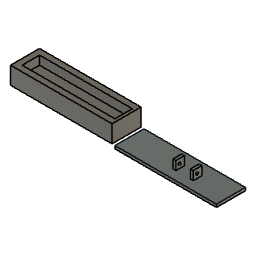
挂灯母 v1 (Autodesk Fusion 360 design; units mm, degrees)
Autodesk Fusion 360 part; units mm, degrees
note: some values were not read from the file. Set by a fixed rule: which face or edge a step refers to.
sketch "草图1" plane through (0, 0, 0) normal (0, 0, 1) x (1, 0, 0)
  line L0 (0, 20) -> (35, 20)
  line L1 (35, 20) -> (35, 10)
  line L2 (35, 10) -> (0, 10)
  line L3 (0, 10) -> (0, 20)
  constraint horizontal L0
  constraint vertical L1
  constraint horizontal L2
  constraint vertical L3
extrude "拉伸1" add sketch "草图1" along normal blind 6 makes body 1
sketch "草图2" plane through (0, 0, 6) normal (0, 0, 1) x (-1, 0, 0)
  line L0 (0, -10) -> (-35, -10)
  line L1 (-35, -10) -> (-35, -20)
  line L2 (-35, -20) -> (0, -20)
  line L3 (0, -20) -> (0, -10)
  line L4 (-34, -12) -> (-2, -12)
  line L5 (-2, -12) -> (-2, -18)
  line L6 (-2, -18) -> (-34, -18)
  line L7 (-34, -18) -> (-34, -12)
  constraint horizontal L4
  constraint vertical L5
  constraint horizontal L6
  constraint vertical L7
sketch "草图3" plane through (0, 0, 6) normal (0, 0, 1) x (1, 0, 0)
extrude "拉伸2" cut sketch "草图2" against normal blind 3 contours L4 L5 L6 L7 bodies 1
shell "抽壳1" thickness 2 removed faces 1 at (11.6667, 16.6667, 0) on bodies 1
extrude "拉伸3" cut 1 faces at (12.3333, 16, 1) along direction (0, 0, 1) blind 1 on bodies 1 bodies 1
sketch "草图4" plane through (0, 0, 0) normal (0, 0, -1) x (1, 0, 0)
  line L0 (2, -12) -> (33, -12)
  line L1 (33, -12) -> (33, -18)
  line L2 (33, -18) -> (2, -18)
  line L3 (2, -18) -> (2, -12)
  line L4 (35, -10) -> (0, -10)
  line L5 (0, -10) -> (0, -20)
  line L6 (0, -20) -> (35, -20)
  line L7 (35, -20) -> (35, -10)
  line L8 (0, -10) -> (35, -10)
  line L9 (35, -10) -> (35, -20)
  line L10 (35, -20) -> (0, -20)
  line L11 (0, -20) -> (0, -10)
  constraint horizontal L8
  constraint vertical L9
  constraint horizontal L10
  constraint vertical L11
  constraint coincident L6.end L7.start
  constraint coincident L4.end L5.start
move_body "移动1" bodies 1 to x (1, 0, 0) y (0, 1, 0) z (0, 0, 1) at (-36, 0, 0)
extrude "拉伸4" add sketch "草图4" along normal blind 1 separate body contours L0 L1 L2 L3 | L4 L5 L6 L7 L8 L9 L10 L11 makes body 2
sketch "草图5" plane through (0, 0, 0) normal (0, 0, 1) x (-1, 0, 0)
  line L0 (-35, -20) -> (0, -20)
  line L1 (0, -20) -> (0, -10)
  line L2 (0, -10) -> (-35, -10)
  line L3 (-35, -10) -> (-35, -20)
sketch "草图6" plane through (0, 0, 0) normal (0, 0, 1) x (1, 0, 0)
sketch "草图7" plane through (0, 0, 0) normal (0, 0, 1) x (-1, 0, 0)
  line L0 (-24, -13) -> (-23, -13)
  line L1 (-23, -13) -> (-23, -16)
  line L2 (-23, -16) -> (-24, -16)
  line L3 (-24, -16) -> (-24, -13)
  line L4 (-18, -13) -> (-17, -13)
  line L5 (-17, -13) -> (-17, -16)
  line L6 (-17, -16) -> (-18, -16)
  line L7 (-18, -16) -> (-18, -13)
  constraint horizontal L0
  constraint vertical L1
  constraint horizontal L2
  constraint vertical L3
  constraint horizontal L4
  constraint vertical L5
  constraint horizontal L6
  constraint vertical L7
extrude "拉伸5" add sketch "草图7" along normal blind 3 bodies 2
hole "孔1" at (24, 14.323, 1.4488) direction (-1, 0, 0) diameter 1 depth 10 tip angle 118 bodies 2
